Autodesk Fusion 360 part; units mm, degrees
(part 5 of 7)
extrude "Optical screw head (1)" add sketch "Optical screw head profile (1)" against normal blind 1.65 separate body makes body 166 in component "REF M3 screws"
ref_plane "WorkPlane12" through (0, 0, -3.075) normal (0, 0, 1) x (1, 0, 0) in component "REF M3 screws"
sketch "Optical screw shaft profile (1)" plane through (0, 0, -3.075) normal (0, 0, 1) x (1, 0, 0) in component "REF M3 screws"
  circle A0 centre (60, 54) radius 1.5
  dimension "d1280" = 3
  measures "d1280" diameter of A0
extrude "Optical screw shaft (1)" add sketch "Optical screw shaft profile (1)" against normal blind 6 separate body makes body 167 in component "REF M3 screws"
ref_plane "WorkPlane13" through (0, 0, -7.75) normal (0, 0, 1) x (1, 0, 0) in component "REF M3 screws"
sketch "Yoke screw head profile" plane through (0, 0, -7.75) normal (0, 0, 1) x (1, 0, 0) in component "REF M3 screws"
  circle A0 centre (35, 38) radius 2.85
  dimension "d1285" = 5.7
  measures "d1285" diameter of A0
extrude "Yoke screw head" add sketch "Yoke screw head profile" against normal blind 1.65 separate body makes body 168 in component "REF M3 screws"
ref_plane "WorkPlane14" through (0, 0, -9.4) normal (0, 0, 1) x (1, 0, 0) in component "REF M3 screws"
sketch "Yoke screw shaft profile" plane through (0, 0, -9.4) normal (0, 0, 1) x (1, 0, 0) in component "REF M3 screws"
  circle A0 centre (35, 38) radius 1.5
  dimension "d1290" = 3
  measures "d1290" diameter of A0
extrude "Yoke screw shaft" add sketch "Yoke screw shaft profile" against normal blind 8 separate body makes body 169 in component "REF M3 screws"
ref_plane "WorkPlane15" through (0, 0, -7.75) normal (0, 0, 1) x (1, 0, 0) in component "REF M3 screws"
sketch "Yoke screw head profile (1)" plane through (0, 0, -7.75) normal (0, 0, 1) x (1, 0, 0) in component "REF M3 screws"
  circle A0 centre (103, 38) radius 2.85
  dimension "d1295" = 5.7
  measures "d1295" diameter of A0
extrude "Yoke screw head (1)" add sketch "Yoke screw head profile (1)" against normal blind 1.65 separate body makes body 170 in component "REF M3 screws"
ref_plane "WorkPlane16" through (0, 0, -9.4) normal (0, 0, 1) x (1, 0, 0) in component "REF M3 screws"
sketch "Yoke screw shaft profile (1)" plane through (0, 0, -9.4) normal (0, 0, 1) x (1, 0, 0) in component "REF M3 screws"
  circle A0 centre (103, 38) radius 1.5
  dimension "d1300" = 3
  measures "d1300" diameter of A0
extrude "Yoke screw shaft (1)" add sketch "Yoke screw shaft profile (1)" against normal blind 8 separate body makes body 171 in component "REF M3 screws"
ref_plane "WorkPlane1" through (0, 0, -24.9) normal (0, 0, 1) x (1, 0, 0) in component "REF M3 nuts"
sketch "Nut hex" plane through (0, 0, -24.9) normal (0, 0, 1) x (1, 0, 0) in component "REF M3 nuts"
  line L0 (9.1754, 6) -> (7.5877, 8.75)
  line L1 (7.5877, 8.75) -> (4.4123, 8.75)
  line L2 (4.4123, 8.75) -> (2.8246, 6)
  line L3 (2.8246, 6) -> (4.4123, 3.25)
  line L4 (4.4123, 3.25) -> (7.5877, 3.25)
  line L5 (7.5877, 3.25) -> (9.1754, 6)
extrude "M3 nut" add sketch "Nut hex" against normal blind 2.4 separate body makes body 172 in component "REF M3 nuts"
ref_plane "WorkPlane2" through (0, 0, -24.89) normal (0, 0, 1) x (1, 0, 0) in component "REF M3 nuts"
sketch "Reference thread clearance profile" plane through (0, 0, -24.89) normal (0, 0, 1) x (1, 0, 0) in component "REF M3 nuts"
  circle A0 centre (6, 6) radius 1.575
  dimension "d1309" = 3.15
  measures "d1309" diameter of A0
extrude "Reference thread clearance" cut sketch "Reference thread clearance profile" against normal blind 2.42 bodies 172 in component "REF M3 nuts"
ref_plane "WorkPlane3" through (0, 0, -24.9) normal (0, 0, 1) x (1, 0, 0) in component "REF M3 nuts"
sketch "Nut hex (1)" plane through (0, 0, -24.9) normal (0, 0, 1) x (1, 0, 0) in component "REF M3 nuts"
  line L0 (117.1754, 6) -> (115.5877, 8.75)
  line L1 (115.5877, 8.75) -> (112.4123, 8.75)
  line L2 (112.4123, 8.75) -> (110.8246, 6)
  line L3 (110.8246, 6) -> (112.4123, 3.25)
  line L4 (112.4123, 3.25) -> (115.5877, 3.25)
  line L5 (115.5877, 3.25) -> (117.1754, 6)
extrude "M3 nut (1)" add sketch "Nut hex (1)" against normal blind 2.4 separate body makes body 173 in component "REF M3 nuts"
ref_plane "WorkPlane4" through (0, 0, -24.89) normal (0, 0, 1) x (1, 0, 0) in component "REF M3 nuts"
sketch "Reference thread clearance profile (1)" plane through (0, 0, -24.89) normal (0, 0, 1) x (1, 0, 0) in component "REF M3 nuts"
  circle A0 centre (114, 6) radius 1.575
  dimension "d1318" = 3.15
  measures "d1318" diameter of A0
extrude "Reference thread clearance (1)" cut sketch "Reference thread clearance profile (1)" against normal blind 2.42 bodies 172 173 in component "REF M3 nuts"
ref_plane "WorkPlane5" through (0, 0, -24.9) normal (0, 0, 1) x (1, 0, 0) in component "REF M3 nuts"
sketch "Nut hex (2)" plane through (0, 0, -24.9) normal (0, 0, 1) x (1, 0, 0) in component "REF M3 nuts"
  line L0 (9.1754, 54) -> (7.5877, 56.75)
  line L1 (7.5877, 56.75) -> (4.4123, 56.75)
  line L2 (4.4123, 56.75) -> (2.8246, 54)
  line L3 (2.8246, 54) -> (4.4123, 51.25)
  line L4 (4.4123, 51.25) -> (7.5877, 51.25)
  line L5 (7.5877, 51.25) -> (9.1754, 54)
extrude "M3 nut (2)" add sketch "Nut hex (2)" against normal blind 2.4 separate body makes body 174 in component "REF M3 nuts"
ref_plane "WorkPlane6" through (0, 0, -24.89) normal (0, 0, 1) x (1, 0, 0) in component "REF M3 nuts"
sketch "Reference thread clearance profile (2)" plane through (0, 0, -24.89) normal (0, 0, 1) x (1, 0, 0) in component "REF M3 nuts"
  circle A0 centre (6, 54) radius 1.575
  dimension "d1327" = 3.15
  measures "d1327" diameter of A0
extrude "Reference thread clearance (2)" cut sketch "Reference thread clearance profile (2)" against normal blind 2.42 bodies 172 173 174 in component "REF M3 nuts"
ref_plane "WorkPlane7" through (0, 0, -24.9) normal (0, 0, 1) x (1, 0, 0) in component "REF M3 nuts"
sketch "Nut hex (3)" plane through (0, 0, -24.9) normal (0, 0, 1) x (1, 0, 0) in component "REF M3 nuts"
  line L0 (99.1754, 54) -> (97.5877, 56.75)
  line L1 (97.5877, 56.75) -> (94.4123, 56.75)
  line L2 (94.4123, 56.75) -> (92.8246, 54)
  line L3 (92.8246, 54) -> (94.4123, 51.25)
  line L4 (94.4123, 51.25) -> (97.5877, 51.25)
  line L5 (97.5877, 51.25) -> (99.1754, 54)
extrude "M3 nut (3)" add sketch "Nut hex (3)" against normal blind 2.4 separate body makes body 175 in component "REF M3 nuts"
ref_plane "WorkPlane8" through (0, 0, -24.89) normal (0, 0, 1) x (1, 0, 0) in component "REF M3 nuts"
sketch "Reference thread clearance profile (3)" plane through (0, 0, -24.89) normal (0, 0, 1) x (1, 0, 0) in component "REF M3 nuts"
  circle A0 centre (96, 54) radius 1.575
  dimension "d1336" = 3.15
  measures "d1336" diameter of A0
extrude "Reference thread clearance (3)" cut sketch "Reference thread clearance profile (3)" against normal blind 2.42 bodies 172 173 174 175 in component "REF M3 nuts"
ref_plane "WorkPlane9" through (0, 0, -3.3) normal (0, 0, 1) x (1, 0, 0) in component "REF M3 nuts"
sketch "Nut hex (4)" plane through (0, 0, -3.3) normal (0, 0, 1) x (1, 0, 0) in component "REF M3 nuts"
  line L0 (63.1754, 6) -> (61.5877, 8.75)
  line L1 (61.5877, 8.75) -> (58.4123, 8.75)
  line L2 (58.4123, 8.75) -> (56.8246, 6)
  line L3 (56.8246, 6) -> (58.4123, 3.25)
  line L4 (58.4123, 3.25) -> (61.5877, 3.25)
  line L5 (61.5877, 3.25) -> (63.1754, 6)
extrude "M3 nut (4)" add sketch "Nut hex (4)" against normal blind 2.4 separate body makes body 176 in component "REF M3 nuts"
ref_plane "WorkPlane10" through (0, 0, -3.29) normal (0, 0, 1) x (1, 0, 0) in component "REF M3 nuts"
sketch "Reference thread clearance profile (4)" plane through (0, 0, -3.29) normal (0, 0, 1) x (1, 0, 0) in component "REF M3 nuts"
  circle A0 centre (60, 6) radius 1.575
  dimension "d1345" = 3.15
  measures "d1345" diameter of A0
extrude "Reference thread clearance (4)" cut sketch "Reference thread clearance profile (4)" against normal blind 2.42 bodies 172 173 174 175 176 in component "REF M3 nuts"
ref_plane "WorkPlane11" through (0, 0, -3.3) normal (0, 0, 1) x (1, 0, 0) in component "REF M3 nuts"
sketch "Nut hex (5)" plane through (0, 0, -3.3) normal (0, 0, 1) x (1, 0, 0) in component "REF M3 nuts"
  line L0 (63.1754, 54) -> (61.5877, 56.75)
  line L1 (61.5877, 56.75) -> (58.4123, 56.75)
  line L2 (58.4123, 56.75) -> (56.8246, 54)
  line L3 (56.8246, 54) -> (58.4123, 51.25)
  line L4 (58.4123, 51.25) -> (61.5877, 51.25)
  line L5 (61.5877, 51.25) -> (63.1754, 54)
extrude "M3 nut (5)" add sketch "Nut hex (5)" against normal blind 2.4 separate body makes body 177 in component "REF M3 nuts"
ref_plane "WorkPlane12" through (0, 0, -3.29) normal (0, 0, 1) x (1, 0, 0) in component "REF M3 nuts"
sketch "Reference thread clearance profile (5)" plane through (0, 0, -3.29) normal (0, 0, 1) x (1, 0, 0) in component "REF M3 nuts"
  circle A0 centre (60, 54) radius 1.575
  dimension "d1354" = 3.15
  measures "d1354" diameter of A0
extrude "Reference thread clearance (5)" cut sketch "Reference thread clearance profile (5)" against normal blind 2.42 bodies 172 173 174 175 176 177 in component "REF M3 nuts"
ref_plane "WorkPlane13" through (0, 0, -13.9) normal (0, 0, 1) x (1, 0, 0) in component "REF M3 nuts"
sketch "Nut hex (6)" plane through (0, 0, -13.9) normal (0, 0, 1) x (1, 0, 0) in component "REF M3 nuts"
  line L0 (38.1754, 38) -> (36.5877, 40.75)
  line L1 (36.5877, 40.75) -> (33.4123, 40.75)
  line L2 (33.4123, 40.75) -> (31.8246, 38)
  line L3 (31.8246, 38) -> (33.4123, 35.25)
  line L4 (33.4123, 35.25) -> (36.5877, 35.25)
  line L5 (36.5877, 35.25) -> (38.1754, 38)
extrude "M3 nut (6)" add sketch "Nut hex (6)" against normal blind 2.4 separate body makes body 178 in component "REF M3 nuts"
ref_plane "WorkPlane14" through (0, 0, -13.89) normal (0, 0, 1) x (1, 0, 0) in component "REF M3 nuts"
sketch "Reference thread clearance profile (6)" plane through (0, 0, -13.89) normal (0, 0, 1) x (1, 0, 0) in component "REF M3 nuts"
  circle A0 centre (35, 38) radius 1.575
  dimension "d1363" = 3.15
  measures "d1363" diameter of A0
extrude "Reference thread clearance (6)" cut sketch "Reference thread clearance profile (6)" against normal blind 2.42 bodies 172 173 174 175 176 177 178 in component "REF M3 nuts"
ref_plane "WorkPlane15" through (0, 0, -13.9) normal (0, 0, 1) x (1, 0, 0) in component "REF M3 nuts"
sketch "Nut hex (7)" plane through (0, 0, -13.9) normal (0, 0, 1) x (1, 0, 0) in component "REF M3 nuts"
  line L0 (106.1754, 38) -> (104.5877, 40.75)
  line L1 (104.5877, 40.75) -> (101.4123, 40.75)
  line L2 (101.4123, 40.75) -> (99.8246, 38)
  line L3 (99.8246, 38) -> (101.4123, 35.25)
  line L4 (101.4123, 35.25) -> (104.5877, 35.25)
  line L5 (104.5877, 35.25) -> (106.1754, 38)
extrude "M3 nut (7)" add sketch "Nut hex (7)" against normal blind 2.4 separate body makes body 179 in component "REF M3 nuts"
ref_plane "WorkPlane16" through (0, 0, -13.89) normal (0, 0, 1) x (1, 0, 0) in component "REF M3 nuts"
sketch "Reference thread clearance profile (7)" plane through (0, 0, -13.89) normal (0, 0, 1) x (1, 0, 0) in component "REF M3 nuts"
  circle A0 centre (103, 38) radius 1.575
  dimension "d1372" = 3.15
  measures "d1372" diameter of A0
extrude "Reference thread clearance (7)" cut sketch "Reference thread clearance profile (7)" against normal blind 2.42 bodies 172 173 174 175 176 177 178 179 in component "REF M3 nuts"
ref_plane "WorkPlane67" through (0, 0, -9.48) normal (0, 0, 1) x (1, 0, 0) in component "05 Rear electronics housing"
sketch "Charger straight assembly notch profile" plane through (0, 0, -9.48) normal (0, 0, 1) x (1, 0, 0) in component "05 Rear electronics housing"
  line L0 (14.8, 57.4) -> (28.2, 57.4)
  line L1 (28.2, 57.4) -> (28.2, 60.2)
  line L2 (28.2, 60.2) -> (14.8, 60.2)
  line L3 (14.8, 60.2) -> (14.8, 57.4)
  dimension "d1377" = 13.4
  dimension "d1378" = 2.8
  measures "d1377" horizontal distance of L0.start L0.end
  measures "d1378" vertical distance of L0.end L1.end
extrude "Charger straight assembly notch" cut sketch "Charger straight assembly notch profile" against normal blind 11.03 bodies 66 in component "05 Rear electronics housing"
ref_plane "WorkPlane53" through (0, 0, -9.15) normal (0, 0, 1) x (1, 0, 0) in component "01 Front optical bezel"
sketch "Charger yoke cap seam clearance profile" plane through (0, 0, -9.15) normal (0, 0, 1) x (1, 0, 0) in component "01 Front optical bezel"
  line L0 (14.8, 57.4) -> (28.2, 57.4)
  line L1 (28.2, 57.4) -> (28.2, 60.2)
  line L2 (28.2, 60.2) -> (14.8, 60.2)
  line L3 (14.8, 60.2) -> (14.8, 57.4)
  dimension "d1383" = 13.4
  dimension "d1384" = 2.8
  measures "d1383" horizontal distance of L0.start L0.end
  measures "d1384" vertical distance of L0.end L1.end
extrude "Charger yoke cap seam clearance" cut sketch "Charger yoke cap seam clearance profile" against normal blind 0.5 bodies 1 in component "01 Front optical bezel"
ref_plane "WorkPlane68" through (0, 0, -9.48) normal (0, 0, 1) x (1, 0, 0) in component "05 Rear electronics housing"
sketch "XIAO straight assembly notch profile" plane through (0, 0, -9.48) normal (0, 0, 1) x (1, 0, 0) in component "05 Rear electronics housing"
  line L0 (110.4, 57) -> (117.5, 57)
  line L1 (117.5, 57) -> (117.5, 60.2)
  line L2 (117.5, 60.2) -> (110.4, 60.2)
  line L3 (110.4, 60.2) -> (110.4, 57)
  dimension "d1389" = 7.1
  dimension "d1390" = 3.2
  measures "d1389" horizontal distance of L0.start L0.end
  measures "d1390" vertical distance of L0.end L1.end
extrude "XIAO straight assembly notch" cut sketch "XIAO straight assembly notch profile" against normal blind 8.53 bodies 66 in component "05 Rear electronics housing"
ref_plane "WorkPlane54" through (0, 0, -9.15) normal (0, 0, 1) x (1, 0, 0) in component "01 Front optical bezel"
sketch "XIAO yoke cap seam clearance profile" plane through (0, 0, -9.15) normal (0, 0, 1) x (1, 0, 0) in component "01 Front optical bezel"
  line L0 (110.4, 57.4) -> (117.5, 57.4)
  line L1 (117.5, 57.4) -> (117.5, 60.2)
  line L2 (117.5, 60.2) -> (110.4, 60.2)
  line L3 (110.4, 60.2) -> (110.4, 57.4)
  dimension "d1395" = 7.1
  dimension "d1396" = 2.8
  measures "d1395" horizontal distance of L0.start L0.end
  measures "d1396" vertical distance of L0.end L1.end
extrude "XIAO yoke cap seam clearance" cut sketch "XIAO yoke cap seam clearance profile" against normal blind 0.5 bodies 1 in component "01 Front optical bezel"
ref_plane "WorkPlane69" through (0, 0, -9.48) normal (0, 0, 1) x (1, 0, 0) in component "05 Rear electronics housing"
sketch "Slider straight assembly notch profile" plane through (0, 0, -9.48) normal (0, 0, 1) x (1, 0, 0) in component "05 Rear electronics housing"
  line L0 (55.25, 57.4) -> (64.75, 57.4)
  line L1 (64.75, 57.4) -> (64.75, 60.2)
  line L2 (64.75, 60.2) -> (55.25, 60.2)
  line L3 (55.25, 60.2) -> (55.25, 57.4)
  dimension "d1401" = 9.5
  dimension "d1402" = 2.8
  measures "d1401" horizontal distance of L0.start L0.end
  measures "d1402" vertical distance of L0.end L1.end
extrude "Slider straight assembly notch" cut sketch "Slider straight assembly notch profile" against normal blind 11.63 bodies 66 in component "05 Rear electronics housing"
ref_plane "WorkPlane55" through (0, 0, -9.15) normal (0, 0, 1) x (1, 0, 0) in component "01 Front optical bezel"
sketch "Slider yoke cap seam clearance profile" plane through (0, 0, -9.15) normal (0, 0, 1) x (1, 0, 0) in component "01 Front optical bezel"
  line L0 (55.25, 57.4) -> (64.75, 57.4)
  line L1 (64.75, 57.4) -> (64.75, 60.2)
  line L2 (64.75, 60.2) -> (55.25, 60.2)
  line L3 (55.25, 60.2) -> (55.25, 57.4)
  dimension "d1407" = 9.5
  dimension "d1408" = 2.8
  measures "d1407" horizontal distance of L0.start L0.end
  measures "d1408" vertical distance of L0.end L1.end
extrude "Slider yoke cap seam clearance" cut sketch "Slider yoke cap seam clearance profile" against normal blind 0.5 bodies 1 in component "01 Front optical bezel"
ref_plane "WorkPlane70" through (0, 0, -9.48) normal (0, 0, 1) x (1, 0, 0) in component "05 Rear electronics housing"
sketch "Reset front insertion notch profile" plane through (0, 0, -9.48) normal (0, 0, 1) x (1, 0, 0) in component "05 Rear electronics housing"
  line L0 (116.1, 52.55) -> (120.2, 52.55)
  line L1 (120.2, 52.55) -> (120.2, 56.85)
  line L2 (120.2, 56.85) -> (116.1, 56.85)
  line L3 (116.1, 56.85) -> (116.1, 52.55)
  dimension "d1413" = 4.1
  dimension "d1414" = 4.3
  measures "d1413" horizontal distance of L0.start L0.end
  measures "d1414" vertical distance of L0.end L1.end
extrude "Reset front insertion notch" cut sketch "Reset front insertion notch profile" against normal blind 4.53 bodies 66 in component "05 Rear electronics housing"
ref_plane "WorkPlane56" through (0, 0, -9.15) normal (0, 0, 1) x (1, 0, 0) in component "01 Front optical bezel"
sketch "Reset cap seam clearance profile" plane through (0, 0, -9.15) normal (0, 0, 1) x (1, 0, 0) in component "01 Front optical bezel"
  line L0 (116.1, 52.55) -> (120.2, 52.55)
  line L1 (120.2, 52.55) -> (120.2, 56.85)
  line L2 (120.2, 56.85) -> (116.1, 56.85)
  line L3 (116.1, 56.85) -> (116.1, 52.55)
  dimension "d1419" = 4.1
  dimension "d1420" = 4.3
  measures "d1419" horizontal distance of L0.start L0.end
  measures "d1420" vertical distance of L0.end L1.end
extrude "Reset cap seam clearance" cut sketch "Reset cap seam clearance profile" against normal blind 0.5 bodies 1 in component "01 Front optical bezel"
ref_plane "WorkPlane71" through (0, 0, -23.09) normal (0, 0, 1) x (1, 0, 0) in component "05 Rear electronics housing"
sketch "DPDT seat to slider clearance profile" plane through (0, 0, -23.09) normal (0, 0, 1) x (1, 0, 0) in component "05 Rear electronics housing"
  line L0 (55.44, 52.15) -> (64.56, 52.15)
  line L1 (64.56, 52.15) -> (64.56, 52.46)
  line L2 (64.56, 52.46) -> (55.44, 52.46)
  line L3 (55.44, 52.46) -> (55.44, 52.15)
  dimension "d1425" = 9.12
  dimension "d1426" = 0.31
  measures "d1425" horizontal distance of L0.start L0.end
  measures "d1426" vertical distance of L0.end L1.end
extrude "DPDT seat to slider clearance" cut sketch "DPDT seat to slider clearance profile" against normal blind 8.62 bodies 66 in component "05 Rear electronics housing"
ref_plane "WorkPlane25" through (0, 0, -9.4) normal (0, 0, 1) x (1, 0, 0) in component "06 Electronics retaining yoke"
sketch "Charger port cap arm profile" plane through (0, 0, -9.4) normal (0, 0, 1) x (1, 0, 0) in component "06 Electronics retaining yoke"
  line L0 (13.1, 52) -> (15.1, 52)
  line L1 (15.1, 52) -> (15.1, 57.4)
  line L2 (15.1, 57.4) -> (13.1, 57.4)
  line L3 (13.1, 57.4) -> (13.1, 52)
  dimension "d1431" = 2
  dimension "d1432" = 5.4
  measures "d1431" horizontal distance of L0.start L0.end
  measures "d1432" vertical distance of L0.end L1.end
extrude "Charger port cap arm" add sketch "Charger port cap arm profile" against normal blind 2 separate body makes body 180 in component "06 Electronics retaining yoke"
ref_plane "WorkPlane26" through (0, 0, -9.4) normal (0, 0, 1) x (1, 0, 0) in component "06 Electronics retaining yoke"
sketch "Charger port cap arm profile (1)" plane through (0, 0, -9.4) normal (0, 0, 1) x (1, 0, 0) in component "06 Electronics retaining yoke"
  line L0 (26.9, 52) -> (28.9, 52)
  line L1 (28.9, 52) -> (28.9, 57.4)
  line L2 (28.9, 57.4) -> (26.9, 57.4)
  line L3 (26.9, 57.4) -> (26.9, 52)
  dimension "d1437" = 2
  dimension "d1438" = 5.4
  measures "d1437" horizontal distance of L0.start L0.end
  measures "d1438" vertical distance of L0.end L1.end
extrude "Charger port cap arm (1)" add sketch "Charger port cap arm profile (1)" against normal blind 2 separate body makes body 181 in component "06 Electronics retaining yoke"
ref_plane "WorkPlane27" through (0, 0, -9.4) normal (0, 0, 1) x (1, 0, 0) in component "06 Electronics retaining yoke"
sketch "Charger port roof profile" plane through (0, 0, -9.4) normal (0, 0, 1) x (1, 0, 0) in component "06 Electronics retaining yoke"
  line L0 (15.05, 57.15) -> (27.95, 57.15)
  line L1 (27.95, 57.15) -> (27.95, 59.75)
  line L2 (27.95, 59.75) -> (15.05, 59.75)
  line L3 (15.05, 59.75) -> (15.05, 57.15)
  dimension "d1443" = 12.9
  dimension "d1444" = 2.6
  measures "d1443" horizontal distance of L0.start L0.end
  measures "d1444" vertical distance of L0.end L1.end
extrude "Charger port roof" add sketch "Charger port roof profile" against normal blind 8.85 separate body makes body 182 in component "06 Electronics retaining yoke"
ref_plane "WorkPlane28" through (0, 0, -9.4) normal (0, 0, 1) x (1, 0, 0) in component "06 Electronics retaining yoke"
sketch "XIAO port cap arm profile" plane through (0, 0, -9.4) normal (0, 0, 1) x (1, 0, 0) in component "06 Electronics retaining yoke"
  line L0 (108.5, 49) -> (110.8, 49)
  line L1 (110.8, 49) -> (110.8, 57.4)
  line L2 (110.8, 57.4) -> (108.5, 57.4)
  line L3 (108.5, 57.4) -> (108.5, 49)
  dimension "d1449" = 2.3
  dimension "d1450" = 8.4
  measures "d1449" horizontal distance of L0.start L0.end
  measures "d1450" vertical distance of L0.end L1.end
extrude "XIAO port cap arm" add sketch "XIAO port cap arm profile" against normal blind 2 separate body makes body 183 in component "06 Electronics retaining yoke"
ref_plane "WorkPlane29" through (0, 0, -9.4) normal (0, 0, 1) x (1, 0, 0) in component "06 Electronics retaining yoke"
sketch "XIAO port roof profile" plane through (0, 0, -9.4) normal (0, 0, 1) x (1, 0, 0) in component "06 Electronics retaining yoke"
  line L0 (110.65, 57.15) -> (117.25, 57.15)
  line L1 (117.25, 57.15) -> (117.25, 59.75)
  line L2 (117.25, 59.75) -> (110.65, 59.75)
  line L3 (110.65, 59.75) -> (110.65, 57.15)
  dimension "d1455" = 6.6
  dimension "d1456" = 2.6
  measures "d1455" horizontal distance of L0.start L0.end
  measures "d1456" vertical distance of L0.end L1.end
extrude "XIAO port roof" add sketch "XIAO port roof profile" against normal blind 6.85 separate body makes body 184 in component "06 Electronics retaining yoke"
ref_plane "WorkPlane30" through (0, 0, -9.4) normal (0, 0, 1) x (1, 0, 0) in component "06 Electronics retaining yoke"
sketch "Slider cap arm profile" plane through (0, 0, -9.4) normal (0, 0, 1) x (1, 0, 0) in component "06 Electronics retaining yoke"
  line L0 (55.5, 51) -> (56.9, 51)
  line L1 (56.9, 51) -> (56.9, 57.4)
  line L2 (56.9, 57.4) -> (55.5, 57.4)
  line L3 (55.5, 57.4) -> (55.5, 51)
  dimension "d1461" = 1.4
  dimension "d1462" = 6.4
  measures "d1461" horizontal distance of L0.start L0.end
  measures "d1462" vertical distance of L0.end L1.end
extrude "Slider cap arm" add sketch "Slider cap arm profile" against normal blind 2 separate body makes body 185 in component "06 Electronics retaining yoke"
ref_plane "WorkPlane31" through (0, 0, -9.4) normal (0, 0, 1) x (1, 0, 0) in component "06 Electronics retaining yoke"
sketch "Slider cap arm profile (1)" plane through (0, 0, -9.4) normal (0, 0, 1) x (1, 0, 0) in component "06 Electronics retaining yoke"
  line L0 (63.1, 51) -> (64.5, 51)
  line L1 (64.5, 51) -> (64.5, 57.4)
  line L2 (64.5, 57.4) -> (63.1, 57.4)
  line L3 (63.1, 57.4) -> (63.1, 51)
  dimension "d1467" = 1.4
  dimension "d1468" = 6.4
  measures "d1467" horizontal distance of L0.start L0.end
  measures "d1468" vertical distance of L0.end L1.end
extrude "Slider cap arm (1)" add sketch "Slider cap arm profile (1)" against normal blind 2 separate body makes body 186 in component "06 Electronics retaining yoke"
ref_plane "WorkPlane32" through (0, 0, -9.4) normal (0, 0, 1) x (1, 0, 0) in component "06 Electronics retaining yoke"
sketch "Slider guide roof profile" plane through (0, 0, -9.4) normal (0, 0, 1) x (1, 0, 0) in component "06 Electronics retaining yoke"
  line L0 (55.5, 57.15) -> (64.5, 57.15)
  line L1 (64.5, 57.15) -> (64.5, 59.75)
  line L2 (64.5, 59.75) -> (55.5, 59.75)
  line L3 (55.5, 59.75) -> (55.5, 57.15)
  dimension "d1473" = 9
  dimension "d1474" = 2.6
  measures "d1473" horizontal distance of L0.start L0.end
  measures "d1474" vertical distance of L0.end L1.end
extrude "Slider guide roof" add sketch "Slider guide roof profile" against normal blind 8.85 separate body makes body 187 in component "06 Electronics retaining yoke"
ref_plane "WorkPlane33" through (0, 0, -9.4) normal (0, 0, 1) x (1, 0, 0) in component "06 Electronics retaining yoke"
sketch "Reset cap arm profile" plane through (0, 0, -9.4) normal (0, 0, 1) x (1, 0, 0) in component "06 Electronics retaining yoke"
  line L0 (114.7, 50.8) -> (116.4, 50.8)
  line L1 (116.4, 50.8) -> (116.4, 56.9)
  line L2 (116.4, 56.9) -> (114.7, 56.9)
  line L3 (114.7, 56.9) -> (114.7, 50.8)
  dimension "d1479" = 1.7
  dimension "d1480" = 6.1
  measures "d1479" horizontal distance of L0.start L0.end
  measures "d1480" vertical distance of L0.end L1.end
extrude "Reset cap arm" add sketch "Reset cap arm profile" against normal blind 2 separate body makes body 188 in component "06 Electronics retaining yoke"
ref_plane "WorkPlane34" through (0, 0, -9.4) normal (0, 0, 1) x (1, 0, 0) in component "06 Electronics retaining yoke"
sketch "Reset guide roof profile" plane through (0, 0, -9.4) normal (0, 0, 1) x (1, 0, 0) in component "06 Electronics retaining yoke"
  line L0 (116.2, 52.8) -> (119.75, 52.8)
  line L1 (119.75, 52.8) -> (119.75, 56.6)
  line L2 (119.75, 56.6) -> (116.2, 56.6)
  line L3 (116.2, 56.6) -> (116.2, 52.8)
  dimension "d1485" = 3.55
  dimension "d1486" = 3.8
  measures "d1485" horizontal distance of L0.start L0.end
  measures "d1486" vertical distance of L0.end L1.end
extrude "Reset guide roof" add sketch "Reset guide roof profile" against normal blind 4.3 separate body makes body 189 in component "06 Electronics retaining yoke"
combine "Union manufactured solid (1)'''" operation add target body 106 tool bodies 180 181 182 183 184 185 186 187 188 189 in component "06 Electronics retaining yoke"
ref_plane "WorkPlane35" through (0, 0, -9.4) normal (0, 0, 1) x (1, 0, 0) in component "06 Electronics retaining yoke"
sketch "Charger broad port cap root profile" plane through (0, 0, -9.4) normal (0, 0, 1) x (1, 0, 0) in component "06 Electronics retaining yoke"
  line L0 (13.1, 55.5) -> (28.9, 55.5)
  line L1 (28.9, 55.5) -> (28.9, 57.4)
  line L2 (28.9, 57.4) -> (13.1, 57.4)
  line L3 (13.1, 57.4) -> (13.1, 55.5)
  dimension "d1491" = 15.8
  dimension "d1492" = 1.9
  measures "d1491" horizontal distance of L0.start L0.end
  measures "d1492" vertical distance of L0.end L1.end
extrude "Charger broad port cap root" add sketch "Charger broad port cap root profile" against normal blind 2 separate body makes body 190 in component "06 Electronics retaining yoke"
ref_plane "WorkPlane36" through (0, 0, -9.4) normal (0, 0, 1) x (1, 0, 0) in component "06 Electronics retaining yoke"
sketch "XIAO broad port cap root profile" plane through (0, 0, -9.4) normal (0, 0, 1) x (1, 0, 0) in component "06 Electronics retaining yoke"
  line L0 (108.5, 55.5) -> (117.25, 55.5)
  line L1 (117.25, 55.5) -> (117.25, 57.4)
  line L2 (117.25, 57.4) -> (108.5, 57.4)
  line L3 (108.5, 57.4) -> (108.5, 55.5)
  dimension "d1497" = 8.75
  dimension "d1498" = 1.9
  measures "d1497" horizontal distance of L0.start L0.end
  measures "d1498" vertical distance of L0.end L1.end
extrude "XIAO broad port cap root" add sketch "XIAO broad port cap root profile" against normal blind 2 separate body makes body 191 in component "06 Electronics retaining yoke"
ref_plane "WorkPlane37" through (0, 0, -9.4) normal (0, 0, 1) x (1, 0, 0) in component "06 Electronics retaining yoke"
sketch "Slider broad port cap root profile" plane through (0, 0, -9.4) normal (0, 0, 1) x (1, 0, 0) in component "06 Electronics retaining yoke"
  line L0 (55.5, 55.5) -> (64.5, 55.5)
  line L1 (64.5, 55.5) -> (64.5, 57.4)
  line L2 (64.5, 57.4) -> (55.5, 57.4)
  line L3 (55.5, 57.4) -> (55.5, 55.5)
  dimension "d1503" = 9
  dimension "d1504" = 1.9
  measures "d1503" horizontal distance of L0.start L0.end
  measures "d1504" vertical distance of L0.end L1.end
extrude "Slider broad port cap root" add sketch "Slider broad port cap root profile" against normal blind 2 separate body makes body 192 in component "06 Electronics retaining yoke"
ref_plane "WorkPlane38" through (0, 0, -9.4) normal (0, 0, 1) x (1, 0, 0) in component "06 Electronics retaining yoke"
sketch "Reset broad cap root profile" plane through (0, 0, -9.4) normal (0, 0, 1) x (1, 0, 0) in component "06 Electronics retaining yoke"
  line L0 (114.7, 52.8) -> (117, 52.8)
  line L1 (117, 52.8) -> (117, 56.6)
  line L2 (117, 56.6) -> (114.7, 56.6)
  line L3 (114.7, 56.6) -> (114.7, 52.8)
  dimension "d1509" = 2.3
  dimension "d1510" = 3.8
  measures "d1509" horizontal distance of L0.start L0.end
  measures "d1510" vertical distance of L0.end L1.end
extrude "Reset broad cap root" add sketch "Reset broad cap root profile" against normal blind 2 separate body makes body 193 in component "06 Electronics retaining yoke"
combine "Union manufactured solid (2)''" operation add target body 106 tool bodies 190 191 192 193 in component "06 Electronics retaining yoke"
ref_plane "WorkPlane39" through (0, 0, -9.38) normal (0, 0, 1) x (1, 0, 0) in component "06 Electronics retaining yoke"
sketch "Upper optical screw service clearance profile" plane through (0, 0, -9.38) normal (0, 0, 1) x (1, 0, 0) in component "06 Electronics retaining yoke"
  circle A0 centre (60, 54) radius 3.2
  dimension "d1515" = 6.4
  measures "d1515" diameter of A0
extrude "Upper optical screw service clearance" cut sketch "Upper optical screw service clearance profile" against normal blind 2.04 bodies 106 in component "06 Electronics retaining yoke"
ref_plane "WorkPlane40" through (0, 0, -17.75) normal (0, 0, 1) x (1, 0, 0) in component "06 Electronics retaining yoke"
sketch "Charger cable overmold clearance profile" plane through (0, 0, -17.75) normal (0, 0, 1) x (1, 0, 0) in component "06 Electronics retaining yoke"
  line L0 (15.04, 57.14) -> (27.96, 57.14)
  line L1 (27.96, 57.14) -> (27.96, 59.76)
  line L2 (27.96, 59.76) -> (15.04, 59.76)
  line L3 (15.04, 59.76) -> (15.04, 57.14)
  dimension "d1520" = 12.92
  dimension "d1521" = 2.62
  measures "d1520" horizontal distance of L0.start L0.end
  measures "d1521" vertical distance of L0.end L1.end
extrude "Charger cable overmold clearance" cut sketch "Charger cable overmold clearance profile" against normal blind 0.51 bodies 106 in component "06 Electronics retaining yoke"
ref_plane "WorkPlane41" through (0, 0, -15.2) normal (0, 0, 1) x (1, 0, 0) in component "06 Electronics retaining yoke"
sketch "XIAO cable overmold clearance profile" plane through (0, 0, -15.2) normal (0, 0, 1) x (1, 0, 0) in component "06 Electronics retaining yoke"
  line L0 (110.64, 57.14) -> (117.26, 57.14)
  line L1 (117.26, 57.14) -> (117.26, 59.76)
  line L2 (117.26, 59.76) -> (110.64, 59.76)
  line L3 (110.64, 59.76) -> (110.64, 57.14)
  dimension "d1526" = 6.62
  dimension "d1527" = 2.62
  measures "d1526" horizontal distance of L0.start L0.end
  measures "d1527" vertical distance of L0.end L1.end
extrude "XIAO cable overmold clearance" cut sketch "XIAO cable overmold clearance profile" against normal blind 1.06 bodies 106 in component "06 Electronics retaining yoke"
ref_plane "WorkPlane72" through (0, 0, -27.99) normal (0, 0, 1) x (1, 0, 0) in component "05 Rear electronics housing"
sketch "XIAO cable overmold rear clearance profile" plane through (0, 0, -27.99) normal (0, 0, 1) x (1, 0, 0) in component "05 Rear electronics housing"
  line L0 (110.4, 57.4) -> (117.5, 57.4)
  line L1 (117.5, 57.4) -> (117.5, 60.2)
  line L2 (117.5, 60.2) -> (110.4, 60.2)
  line L3 (110.4, 60.2) -> (110.4, 57.4)
  dimension "d1532" = 7.1
  dimension "d1533" = 2.8
  measures "d1532" horizontal distance of L0.start L0.end
  measures "d1533" vertical distance of L0.end L1.end
extrude "XIAO cable overmold rear clearance" cut sketch "XIAO cable overmold rear clearance profile" against normal blind 1.51 bodies 66 in component "05 Rear electronics housing"
ref_plane "WorkPlane4" through (0, 0, -13.94) normal (0, 0, 1) x (1, 0, 0) in component "07 Captive reset plunger"
sketch "Reset flange to upper port clearance profile" plane through (0, 0, -13.94) normal (0, 0, 1) x (1, 0, 0) in component "07 Captive reset plunger"
  line L0 (115.19, 56.9) -> (116.01, 56.9)
  line L1 (116.01, 56.9) -> (116.01, 57.51)
  line L2 (116.01, 57.51) -> (115.19, 57.51)
  line L3 (115.19, 57.51) -> (115.19, 56.9)
  dimension "d1538" = 0.82
  dimension "d1539" = 0.61
  measures "d1538" horizontal distance of L0.start L0.end
  measures "d1539" vertical distance of L0.end L1.end
extrude "Reset flange to upper port clearance" cut sketch "Reset flange to upper port clearance profile" against normal blind 3.22 bodies 128 in component "07 Captive reset plunger"
ref_plane "WorkPlane73" through (0, 0, -27.1) normal (0, 0, 1) x (1, 0, 0) in component "05 Rear electronics housing"
sketch "Battery fence corner union profile" plane through (0, 0, -27.1) normal (0, 0, 1) x (1, 0, 0) in component "05 Rear electronics housing"
  line L0 (32.4, 32.9) -> (34.1, 32.9)
  line L1 (34.1, 32.9) -> (34.1, 34.6)
  line L2 (34.1, 34.6) -> (32.4, 34.6)
  line L3 (32.4, 34.6) -> (32.4, 32.9)
  dimension "d1544" = 1.7
  dimension "d1545" = 1.7
  measures "d1544" horizontal distance of L0.start L0.end
  measures "d1545" vertical distance of L0.end L1.end
extrude "Battery fence corner union" add sketch "Battery fence corner union profile" against normal blind 4.6 separate body makes body 194 in component "05 Rear electronics housing"
combine "Union manufactured solid (9)" operation add target body 66 tool bodies 194 in component "05 Rear electronics housing"
ref_plane "WorkPlane3" through (0, 0, -4.775) normal (0, 0, 1) x (1, 0, 0) in component "81 Laminate front spacer"
sketch "Inset keyed corner" plane through (0, 0, -4.775) normal (0, 0, 1) x (1, 0, 0) in component "81 Laminate front spacer"
  line L0 (9.5, 47.5) -> (11.6213, 47.5)
  line L1 (11.6213, 47.5) -> (9.5, 45.3787)
  line L2 (9.5, 45.3787) -> (9.5, 47.5)
extrude "Full-width keyed corner" add sketch "Inset keyed corner" against normal blind 0.5 separate body makes body 195 in component "81 Laminate front spacer"
combine "Union manufactured solid'''''''" operation add target body 64 tool bodies 195 in component "81 Laminate front spacer"
ref_plane "WorkPlane3" through (0, 0, -6.875) normal (0, 0, 1) x (1, 0, 0) in component "82 Laminate rear shim"
sketch "Inset keyed corner (2)" plane through (0, 0, -6.875) normal (0, 0, 1) x (1, 0, 0) in component "82 Laminate rear shim"
  line L0 (9.5, 47.5) -> (11.6213, 47.5)
  line L1 (11.6213, 47.5) -> (9.5, 45.3787)
  line L2 (9.5, 45.3787) -> (9.5, 47.5)
extrude "Full-width keyed corner'" add sketch "Inset keyed corner (2)" against normal blind 0.4 separate body makes body 196 in component "82 Laminate rear shim"
combine "Union manufactured solid''''''''" operation add target body 65 tool bodies 196 in component "82 Laminate rear shim"
ref_plane "WorkPlane57" through (0, 0, -3) normal (0, 0, 1) x (1, 0, 0) in component "01 Front optical bezel"
sketch "v21 clearance M3 nut" plane through (0, 0, -3) normal (0, 0, 1) x (1, 0, 0) in component "01 Front optical bezel"
  line L0 (63.4641, 6) -> (61.7321, 9)
  line L1 (61.7321, 9) -> (58.2679, 9)
  line L2 (58.2679, 9) -> (56.5359, 6)
  line L3 (56.5359, 6) -> (58.2679, 3)
  line L4 (58.2679, 3) -> (61.7321, 3)
  line L5 (61.7321, 3) -> (63.4641, 6)
extrude "v21 clearance M3 nut (1)" cut sketch "v21 clearance M3 nut" against normal blind 3 bodies 1 in component "01 Front optical bezel"
ref_plane "WorkPlane58" through (0, 0, -3) normal (0, 0, 1) x (1, 0, 0) in component "01 Front optical bezel"
sketch "v21 nut loading clearance profile" plane through (0, 0, -3) normal (0, 0, 1) x (1, 0, 0) in component "01 Front optical bezel"
  line L0 (60, 3) -> (64.5, 3)
  line L1 (64.5, 3) -> (64.5, 9)
  line L2 (64.5, 9) -> (60, 9)
  line L3 (60, 9) -> (60, 3)
  dimension "d1562" = 4.5
  dimension "d1563" = 6
  measures "d1562" horizontal distance of L0.start L0.end
  measures "d1563" vertical distance of L0.end L1.end
extrude "v21 nut loading clearance" cut sketch "v21 nut loading clearance profile" against normal blind 3 bodies 1 in component "01 Front optical bezel"
ref_plane "WorkPlane59" through (0, 0, -3) normal (0, 0, 1) x (1, 0, 0) in component "01 Front optical bezel"
sketch "v21 clearance M3 nut (1)" plane through (0, 0, -3) normal (0, 0, 1) x (1, 0, 0) in component "01 Front optical bezel"
  line L0 (63.4641, 54) -> (61.7321, 57)
  line L1 (61.7321, 57) -> (58.2679, 57)
  line L2 (58.2679, 57) -> (56.5359, 54)
  line L3 (56.5359, 54) -> (58.2679, 51)
  line L4 (58.2679, 51) -> (61.7321, 51)
  line L5 (61.7321, 51) -> (63.4641, 54)
extrude "v21 clearance M3 nut (2)" cut sketch "v21 clearance M3 nut (1)" against normal blind 3 bodies 1 in component "01 Front optical bezel"
ref_plane "WorkPlane60" through (0, 0, -3) normal (0, 0, 1) x (1, 0, 0) in component "01 Front optical bezel"
sketch "v21 nut loading clearance profile (1)" plane through (0, 0, -3) normal (0, 0, 1) x (1, 0, 0) in component "01 Front optical bezel"
  line L0 (60, 51) -> (64.5, 51)
  line L1 (64.5, 51) -> (64.5, 57)
  line L2 (64.5, 57) -> (60, 57)
  line L3 (60, 57) -> (60, 51)
  dimension "d1572" = 4.5
  dimension "d1573" = 6
  measures "d1572" horizontal distance of L0.start L0.end
  measures "d1573" vertical distance of L0.end L1.end
extrude "v21 nut loading clearance (1)" cut sketch "v21 nut loading clearance profile (1)" against normal blind 3 bodies 1 in component "01 Front optical bezel"
ref_plane "WorkPlane74" through (0, 0, -24.6) normal (0, 0, 1) x (1, 0, 0) in component "05 Rear electronics housing"
sketch "v21 clearance M3 nut (2)" plane through (0, 0, -24.6) normal (0, 0, 1) x (1, 0, 0) in component "05 Rear electronics housing"
  line L0 (9.4641, 6) -> (7.7321, 9)
  line L1 (7.7321, 9) -> (4.2679, 9)
  line L2 (4.2679, 9) -> (2.5359, 6)
  line L3 (2.5359, 6) -> (4.2679, 3)
  line L4 (4.2679, 3) -> (7.7321, 3)
  line L5 (7.7321, 3) -> (9.4641, 6)
extrude "v21 clearance M3 nut (1)'" cut sketch "v21 clearance M3 nut (2)" against normal blind 3 bodies 66 in component "05 Rear electronics housing"
ref_plane "WorkPlane75" through (0, 0, -24.6) normal (0, 0, 1) x (1, 0, 0) in component "05 Rear electronics housing"
sketch "v21 nut loading clearance profile (2)" plane through (0, 0, -24.6) normal (0, 0, 1) x (1, 0, 0) in component "05 Rear electronics housing"
  line L0 (6, 3) -> (10.5, 3)
  line L1 (10.5, 3) -> (10.5, 9)
  line L2 (10.5, 9) -> (6, 9)
  line L3 (6, 9) -> (6, 3)
  dimension "d1582" = 4.5
  dimension "d1583" = 6
  measures "d1582" horizontal distance of L0.start L0.end
  measures "d1583" vertical distance of L0.end L1.end
extrude "v21 nut loading clearance'" cut sketch "v21 nut loading clearance profile (2)" against normal blind 3 bodies 66 in component "05 Rear electronics housing"
ref_plane "WorkPlane76" through (0, 0, -24.6) normal (0, 0, 1) x (1, 0, 0) in component "05 Rear electronics housing"
sketch "v21 clearance M3 nut (1) (2)" plane through (0, 0, -24.6) normal (0, 0, 1) x (1, 0, 0) in component "05 Rear electronics housing"
  line L0 (117.4641, 6) -> (115.7321, 9)
  line L1 (115.7321, 9) -> (112.2679, 9)
  line L2 (112.2679, 9) -> (110.5359, 6)
  line L3 (110.5359, 6) -> (112.2679, 3)
  line L4 (112.2679, 3) -> (115.7321, 3)
  line L5 (115.7321, 3) -> (117.4641, 6)
extrude "v21 clearance M3 nut (2)'" cut sketch "v21 clearance M3 nut (1) (2)" against normal blind 3 bodies 66 in component "05 Rear electronics housing"
ref_plane "WorkPlane77" through (0, 0, -24.6) normal (0, 0, 1) x (1, 0, 0) in component "05 Rear electronics housing"
sketch "v21 nut loading clearance profile (1) (2)" plane through (0, 0, -24.6) normal (0, 0, 1) x (1, 0, 0) in component "05 Rear electronics housing"
  line L0 (109.5, 3) -> (114, 3)
  line L1 (114, 3) -> (114, 9)
  line L2 (114, 9) -> (109.5, 9)
  line L3 (109.5, 9) -> (109.5, 3)
  dimension "d1592" = 4.5
  dimension "d1593" = 6
  measures "d1592" horizontal distance of L0.start L0.end
  measures "d1593" vertical distance of L0.end L1.end
extrude "v21 nut loading clearance (1)'" cut sketch "v21 nut loading clearance profile (1) (2)" against normal blind 3 bodies 66 in component "05 Rear electronics housing"
ref_plane "WorkPlane78" through (0, 0, -24.6) normal (0, 0, 1) x (1, 0, 0) in component "05 Rear electronics housing"
sketch "v21 clearance M3 nut (2) (2)" plane through (0, 0, -24.6) normal (0, 0, 1) x (1, 0, 0) in component "05 Rear electronics housing"
  line L0 (9.4641, 54) -> (7.7321, 57)
  line L1 (7.7321, 57) -> (4.2679, 57)
  line L2 (4.2679, 57) -> (2.5359, 54)
  line L3 (2.5359, 54) -> (4.2679, 51)
  line L4 (4.2679, 51) -> (7.7321, 51)
  line L5 (7.7321, 51) -> (9.4641, 54)
extrude "v21 clearance M3 nut (3)" cut sketch "v21 clearance M3 nut (2) (2)" against normal blind 3 bodies 66 in component "05 Rear electronics housing"
ref_plane "WorkPlane79" through (0, 0, -24.6) normal (0, 0, 1) x (1, 0, 0) in component "05 Rear electronics housing"
sketch "v21 nut loading clearance profile (2) (2)" plane through (0, 0, -24.6) normal (0, 0, 1) x (1, 0, 0) in component "05 Rear electronics housing"
  line L0 (6, 51) -> (10.5, 51)
  line L1 (10.5, 51) -> (10.5, 57)
  line L2 (10.5, 57) -> (6, 57)
  line L3 (6, 57) -> (6, 51)
  dimension "d1602" = 4.5
  dimension "d1603" = 6
  measures "d1602" horizontal distance of L0.start L0.end
  measures "d1603" vertical distance of L0.end L1.end
extrude "v21 nut loading clearance (2)" cut sketch "v21 nut loading clearance profile (2) (2)" against normal blind 3 bodies 66 in component "05 Rear electronics housing"
ref_plane "WorkPlane80" through (0, 0, -24.6) normal (0, 0, 1) x (1, 0, 0) in component "05 Rear electronics housing"
sketch "v21 clearance M3 nut (3)" plane through (0, 0, -24.6) normal (0, 0, 1) x (1, 0, 0) in component "05 Rear electronics housing"
  line L0 (99.4641, 54) -> (97.7321, 57)
  line L1 (97.7321, 57) -> (94.2679, 57)
  line L2 (94.2679, 57) -> (92.5359, 54)
  line L3 (92.5359, 54) -> (94.2679, 51)
  line L4 (94.2679, 51) -> (97.7321, 51)
  line L5 (97.7321, 51) -> (99.4641, 54)
extrude "v21 clearance M3 nut (4)" cut sketch "v21 clearance M3 nut (3)" against normal blind 3 bodies 66 in component "05 Rear electronics housing"
ref_plane "WorkPlane81" through (0, 0, -24.6) normal (0, 0, 1) x (1, 0, 0) in component "05 Rear electronics housing"
sketch "v21 nut loading clearance profile (3)" plane through (0, 0, -24.6) normal (0, 0, 1) x (1, 0, 0) in component "05 Rear electronics housing"
  line L0 (91.5, 51) -> (96, 51)
  line L1 (96, 51) -> (96, 57)
  line L2 (96, 57) -> (91.5, 57)
  line L3 (91.5, 57) -> (91.5, 51)
  dimension "d1612" = 4.5
  dimension "d1613" = 6
  measures "d1612" horizontal distance of L0.start L0.end
  measures "d1613" vertical distance of L0.end L1.end
extrude "v21 nut loading clearance (3)" cut sketch "v21 nut loading clearance profile (3)" against normal blind 3 bodies 66 in component "05 Rear electronics housing"
ref_plane "WorkPlane82" through (0, 0, -13.6) normal (0, 0, 1) x (1, 0, 0) in component "05 Rear electronics housing"
sketch "v21 clearance M3 nut (4)" plane through (0, 0, -13.6) normal (0, 0, 1) x (1, 0, 0) in component "05 Rear electronics housing"
  line L0 (38.4641, 38) -> (36.7321, 41)
  line L1 (36.7321, 41) -> (33.2679, 41)
  line L2 (33.2679, 41) -> (31.5359, 38)
  line L3 (31.5359, 38) -> (33.2679, 35)
  line L4 (33.2679, 35) -> (36.7321, 35)
  line L5 (36.7321, 35) -> (38.4641, 38)
extrude "v21 clearance M3 nut (5)" cut sketch "v21 clearance M3 nut (4)" against normal blind 3 bodies 66 in component "05 Rear electronics housing"
ref_plane "WorkPlane83" through (0, 0, -13.6) normal (0, 0, 1) x (1, 0, 0) in component "05 Rear electronics housing"
sketch "v21 nut loading clearance profile (4)" plane through (0, 0, -13.6) normal (0, 0, 1) x (1, 0, 0) in component "05 Rear electronics housing"
  line L0 (35, 35) -> (39.5, 35)
  line L1 (39.5, 35) -> (39.5, 41)
  line L2 (39.5, 41) -> (35, 41)
  line L3 (35, 41) -> (35, 35)
  dimension "d1622" = 4.5
  dimension "d1623" = 6
  measures "d1622" horizontal distance of L0.start L0.end
  measures "d1623" vertical distance of L0.end L1.end
extrude "v21 nut loading clearance (4)" cut sketch "v21 nut loading clearance profile (4)" against normal blind 3 bodies 66 in component "05 Rear electronics housing"
ref_plane "WorkPlane84" through (0, 0, -13.6) normal (0, 0, 1) x (1, 0, 0) in component "05 Rear electronics housing"
sketch "v21 clearance M3 nut (5)" plane through (0, 0, -13.6) normal (0, 0, 1) x (1, 0, 0) in component "05 Rear electronics housing"
  line L0 (106.4641, 38) -> (104.7321, 41)
  line L1 (104.7321, 41) -> (101.2679, 41)
  line L2 (101.2679, 41) -> (99.5359, 38)
  line L3 (99.5359, 38) -> (101.2679, 35)
  line L4 (101.2679, 35) -> (104.7321, 35)
  line L5 (104.7321, 35) -> (106.4641, 38)
extrude "v21 clearance M3 nut (6)" cut sketch "v21 clearance M3 nut (5)" against normal blind 3 bodies 66 in component "05 Rear electronics housing"
ref_plane "WorkPlane85" through (0, 0, -13.6) normal (0, 0, 1) x (1, 0, 0) in component "05 Rear electronics housing"
sketch "v21 nut loading clearance profile (5)" plane through (0, 0, -13.6) normal (0, 0, 1) x (1, 0, 0) in component "05 Rear electronics housing"
  line L0 (98.5, 35) -> (103, 35)
  line L1 (103, 35) -> (103, 41)
  line L2 (103, 41) -> (98.5, 41)
  line L3 (98.5, 41) -> (98.5, 35)
  dimension "d1632" = 4.5
  dimension "d1633" = 6
  measures "d1632" horizontal distance of L0.start L0.end
  measures "d1633" vertical distance of L0.end L1.end
extrude "v21 nut loading clearance (5)" cut sketch "v21 nut loading clearance profile (5)" against normal blind 3 bodies 66 in component "05 Rear electronics housing"
ref_plane "WorkPlane61" through (0, 0, 0.02) normal (0, 0, 1) x (1, 0, 0) in component "01 Front optical bezel"
sketch "v21 closure screw clearance profile" plane through (0, 0, 0.02) normal (0, 0, 1) x (1, 0, 0) in component "01 Front optical bezel"
  circle A0 centre (6, 6) radius 1.8
  dimension "d1638" = 3.6
  measures "d1638" diameter of A0
extrude "v21 closure screw clearance" cut sketch "v21 closure screw clearance profile" against normal blind 9.6 bodies 1 in component "01 Front optical bezel"
ref_plane "WorkPlane62" through (0, 0, 0.02) normal (0, 0, 1) x (1, 0, 0) in component "01 Front optical bezel"
sketch "v21 socket head clearance profile" plane through (0, 0, 0.02) normal (0, 0, 1) x (1, 0, 0) in component "01 Front optical bezel"
  circle A0 centre (6, 6) radius 3.4
  dimension "d1643" = 6.8
  measures "d1643" diameter of A0
extrude "v21 socket head clearance" cut sketch "v21 socket head clearance profile" against normal blind 3.22 bodies 1 in component "01 Front optical bezel"
ref_plane "WorkPlane86" through (0, 0, -9.48) normal (0, 0, 1) x (1, 0, 0) in component "05 Rear electronics housing"
sketch "v21 closure blind clearance profile" plane through (0, 0, -9.48) normal (0, 0, 1) x (1, 0, 0) in component "05 Rear electronics housing"
  circle A0 centre (6, 6) radius 1.8
  dimension "d1648" = 3.6
  measures "d1648" diameter of A0
extrude "v21 closure blind clearance" cut sketch "v21 closure blind clearance profile" against normal blind 19.72 bodies 66 in component "05 Rear electronics housing"
ref_plane "WorkPlane63" through (0, 0, 0.02) normal (0, 0, 1) x (1, 0, 0) in component "01 Front optical bezel"
sketch "v21 closure screw clearance profile (1)" plane through (0, 0, 0.02) normal (0, 0, 1) x (1, 0, 0) in component "01 Front optical bezel"
  circle A0 centre (114, 6) radius 1.8
  dimension "d1653" = 3.6
  measures "d1653" diameter of A0
extrude "v21 closure screw clearance (1)" cut sketch "v21 closure screw clearance profile (1)" against normal blind 9.6 bodies 1 in component "01 Front optical bezel"
ref_plane "WorkPlane64" through (0, 0, 0.02) normal (0, 0, 1) x (1, 0, 0) in component "01 Front optical bezel"
sketch "v21 socket head clearance profile (1)" plane through (0, 0, 0.02) normal (0, 0, 1) x (1, 0, 0) in component "01 Front optical bezel"
  circle A0 centre (114, 6) radius 3.4
  dimension "d1658" = 6.8
  measures "d1658" diameter of A0
extrude "v21 socket head clearance (1)" cut sketch "v21 socket head clearance profile (1)" against normal blind 3.22 bodies 1 in component "01 Front optical bezel"
ref_plane "WorkPlane87" through (0, 0, -9.48) normal (0, 0, 1) x (1, 0, 0) in component "05 Rear electronics housing"
sketch "v21 closure blind clearance profile (1)" plane through (0, 0, -9.48) normal (0, 0, 1) x (1, 0, 0) in component "05 Rear electronics housing"
  circle A0 centre (114, 6) radius 1.8
  dimension "d1663" = 3.6
  measures "d1663" diameter of A0
extrude "v21 closure blind clearance (1)" cut sketch "v21 closure blind clearance profile (1)" against normal blind 19.72 bodies 66 in component "05 Rear electronics housing"
ref_plane "WorkPlane65" through (0, 0, 0.02) normal (0, 0, 1) x (1, 0, 0) in component "01 Front optical bezel"
sketch "v21 closure screw clearance profile (2)" plane through (0, 0, 0.02) normal (0, 0, 1) x (1, 0, 0) in component "01 Front optical bezel"
  circle A0 centre (6, 54) radius 1.8
  dimension "d1668" = 3.6
  measures "d1668" diameter of A0
extrude "v21 closure screw clearance (2)" cut sketch "v21 closure screw clearance profile (2)" against normal blind 9.6 bodies 1 in component "01 Front optical bezel"
ref_plane "WorkPlane66" through (0, 0, 0.02) normal (0, 0, 1) x (1, 0, 0) in component "01 Front optical bezel"
sketch "v21 socket head clearance profile (2)" plane through (0, 0, 0.02) normal (0, 0, 1) x (1, 0, 0) in component "01 Front optical bezel"
  circle A0 centre (6, 54) radius 3.4
  dimension "d1673" = 6.8
  measures "d1673" diameter of A0